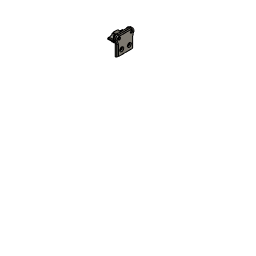
Insert Rig By Sadrita (Autodesk Fusion 360 archive; units mm, degrees)
design "Idler Plate M3"
Autodesk Fusion 360 part; units mm, degrees
sketch "Sketch1" plane through (10, 0, 0) normal (1, 0, 0) x (0, 1, 0)
  line L0 (3.15, 0) -> (10, 0)
  line L1 (10, 0) -> (10, 400)
  line L2 (10, 400) -> (3.15, 400)
  line L3 (3.15, 400) -> (3.15, 0) construction
  line L4 (10, 400) -> (-10, 400) construction
  line L5 (-10, 412) -> (10, 412) construction
  circle A0 centre (6, 412) radius 6
  circle A1 centre (6, 412) radius 2.8
  circle A2 centre (6, 412) radius 1.7
  circle A3 centre (0, 385) radius 2.75
  line L6 (0, 0) -> (0, 505.4699) construction
  line L7 (-10, 464.6221) -> (-10, 380.1585) construction
  circle A4 centre (-26, 412) radius 6
  circle A5 centre (-26, 412) radius 2.8
  circle A6 centre (-26, 412) radius 1.7
  circle A7 centre (6, 412) radius 7.5
  line L8 (10, 400) -> (13.1357, 409.6911)
  line L9 (10, 400) -> (10, 370)
  line L10 (10, 370) -> (-30, 370)
  line L11 (-30, 400) -> (-30, 370)
  line L12 (-30, 400) -> (-33.1357, 409.6911)
  circle A8 centre (-26, 412) radius 7.5
  line L13 (-26, 419.5) -> (6, 419.5)
  circle A9 centre (-20, 385) radius 2.75
  line L14 (2.5, 400) -> (-2.5, 400)
  line L15 (-2.5, 400) -> (-2.5, 370)
  line L16 (-2.5, 370) -> (2.5, 370)
  line L17 (2.5, 370) -> (2.5, 400)
  line L18 (2.5, 400) -> (-2.5, 370) construction
  line L19 (-2.5, 400) -> (2.5, 370) construction
  line L20 (10, 385) -> (-36.1637, 385) construction
  line L21 (-2.5, 391) -> (2.5, 391)
  line L22 (-2.5, 379) -> (2.5, 379)
  line L23 (3.15, 0) -> (10, 0)
  line L24 (10, 0) -> (10, 400)
  line L25 (10, 400) -> (3.15, 400)
  line L26 (3.15, 400) -> (3.15, 0)
  line L27 (-22.5, 370) -> (-22.5, 400)
  line L28 (-22.5, 400) -> (-17.5, 400)
  line L29 (-17.5, 370) -> (-22.5, 370)
  line L30 (-17.5, 400) -> (-17.5, 370)
  line L31 (-17.5, 391) -> (-22.5, 391)
  line L32 (-17.5, 379) -> (-22.5, 379)
  point P0 (6, 394.4653)
  point P1 (0, 385)
  dimension "d22" = 12
  dimension "d33" = 3.4
  dimension "d34" = 12
  dimension "d47" = 5.5
  dimension "d129" = 5.6
  dimension "d166" = 10
  dimension "d167" = 6
  dimension "d168" = 40
  dimension "d169" = 15
  dimension "d170" = 30
  dimension "d171" = 5
  dimension "d172" = 6
  dimension "d173" = 6
  constraint horizontal L4
  constraint coincident L1.end L2.start
  constraint concentric A0 A1
  constraint concentric A1 A2
  constraint vertical A0.centre P0
  constraint coincident L5 A0.centre
  constraint coincident L6.start origin
  constraint perpendicular L5 L6
  constraint vertical L7
  constraint symmetric A0 L7 A4
  constraint symmetric A1 L7 A5
  constraint symmetric A2 L7 A6
  constraint concentric A1 A7
  constraint coincident A7 L8.end
  constraint tangent A7 L8
  constraint coincident L1 L9.end
  constraint perpendicular L4 L9
  constraint perpendicular L9 L10
  constraint symmetric L1.end L7 L11.start
  constraint symmetric L7 A7 A8
  constraint symmetric L7 L8.end L12.end
  constraint symmetric L7 L9.end L10.end
  constraint coincident A8 L13.start
  constraint coincident A7 L13.end
  constraint tangent A7 L13
  constraint perpendicular L6 L13
  constraint coincident P1 L6
  constraint symmetric A3 L7 A9
  constraint horizontal L14
  constraint perpendicular L14 L15
  constraint parallel L14 L16
  constraint parallel L15 L17
  constraint coincident L4 L14.start
  constraint coincident L18 P1
  constraint coincident L19 P1
  constraint coincident P1 A3.centre
  constraint midpoint L9 L20.start
  constraint perpendicular L9 L20
  constraint coincident L10 L16.end
  constraint coincident L15 L21.start
  constraint coincident L17 L21.end
  constraint perpendicular L17 L21
  constraint coincident L15 L22.start
  constraint coincident L17 L22.end
  constraint perpendicular L17 L22
  constraint symmetric L7 L14.start L27.end
  constraint symmetric L7 L14.end L28.end
  constraint symmetric L7 L15.end L29.start
  constraint symmetric L7 L16.end L27.start
  constraint symmetric L7 L21.start L31.start
  constraint symmetric L7 L21.end L31.end
  constraint symmetric L7 L22.start L32.start
  constraint symmetric L7 L22.end L32.end
  measures "d22" diameter of A0
  measures "d33" diameter of A2
  measures "d34" distance of L4 L5
  measures "d47" diameter of A3
  measures "d129" diameter of A1
  measures "d166" distance of L6 L7
  measures "d167" distance of A0.centre L6
  measures "d168" distance of L9.end L10.end
  measures "d169" diameter of A7
  measures "d170" distance of L4 L10
  measures "d171" distance of L15.end L16.end
  measures "d172" distance of P1 L22
  measures "d173" distance of L20 L21
extrude "Extrude1" add sketch "Sketch1" along normal blind 7 contours L1 L2 L9 L10 L24 L25 L26 | L2 A3 A7 L8 L10 L11 L12 A8 L13 A9 L14 L15 L17 L25 L26 L27 L28 L30 | L10 L15 L16 L17 L22 | A3 L15 L17 L22 | A7 | L10 L27 L29 L30 L32 | A9 L27 L30 L32 | A3 L15 L17 L21 | A8 | L14 L15 L17 L21 | A9 L27 L30 L31 | L27 L28 L30 L31 | A0 | A1 | A4 | A5
extrude "Extrude3" add sketch "Sketch1" against normal blind 5.75 contours A0 | A1 | A2 | A4 | A5
extrude "Extrude6" cut sketch "Sketch1" along normal blind 2 from surface at -5.75 contours A0 | A4
extrude "Extrude7" cut sketch "Sketch1" along normal mid plane 28 contours A2
extrude "Extrude11" add sketch "Sketch1" against normal blind 3 contours L10 L15 L16 L17 L22 | L10 L27 L29 L30 L32 | L14 L15 L17 L21 | L27 L28 L30 L31
chamfer "Chamfer2" distance 3 angle 45 4 edges at (7, 0, 391) (7, 0, 379) (7, -20, 391) (7, -20, 379)
chamfer "Chamfer3" distance 1 angle 45 6 edges at (6.25, 0.406, 409.8303) (6.25, 3.3895, 413.0125) (10, 0.406, 409.8303) (10, -31.594, 409.8303) (6.25, -31.594, 409.8303) (6.25, -28.6105, 413.0125)
sketch "Sketch4" plane through (10, 0, 0) normal (-1, 0, 0) x (0, -1, 0)
  circle A0 centre (-6, 412) radius 7
  line L0 (17.5, 400) -> (22.5, 400)
  line L1 (22.5, 400) -> (22.5, 391)
  line L2 (17.5, 391) -> (17.5, 400)
  line L3 (22.5, 379) -> (22.5, 370)
  line L4 (22.5, 370) -> (30, 370)
  line L5 (30, 370) -> (30, 400)
  line L6 (30, 400) -> (33.1357, 409.6911)
  arc A1 (33.1357, 409.6911) -> (26, 419.5) centre (26, 412) ccw
  line L7 (26, 419.5) -> (-6, 419.5)
  arc A2 (-6, 419.5) -> (-13.1357, 409.6911) centre (-6, 412) ccw
  line L8 (-13.1357, 409.6911) -> (-10, 400)
  line L9 (-10, 400) -> (-10, 370)
  line L10 (-10, 370) -> (-2.5, 370)
  line L11 (-2.5, 370) -> (-2.5, 379)
  line L12 (2.5, 379) -> (2.5, 370)
  line L13 (2.5, 370) -> (17.5, 370)
  line L14 (17.5, 370) -> (17.5, 379)
  circle A3 centre (20, 385) radius 2.75
  circle A4 centre (0, 385) radius 2.75
  circle A5 centre (26, 412) radius 7
  line L15 (-10, 400) -> (30, 400)
  line L16 (-10.6471, 402) -> (30.6471, 402)
  circle A6 centre (-6, 412) radius 10
  circle A7 centre (26, 412) radius 10
  line L17 (3.1652, 408) -> (16.8348, 408)
  line L18 (22.5, 391) -> (17.5, 391)
  line L19 (-2.5, 391) -> (-2.5, 400)
  line L20 (-2.5, 400) -> (2.5, 400)
  line L21 (2.5, 400) -> (2.5, 391)
  line L22 (2.5, 391) -> (-2.5, 391)
  line L23 (-2.5, 379) -> (2.5, 379)
  line L24 (17.5, 379) -> (22.5, 379)
  dimension "d2" = 2
  dimension "d3" = 8
  constraint coincident L8.end L9.start
  constraint coincident L5.end L6.start
  constraint coincident L8 L16.start
  constraint coincident L6 L16.end
  constraint parallel L15 L16
  constraint concentric A0 A6
  constraint tangent L16 A6
  constraint concentric A1 A7
  constraint tangent L16 A7
  constraint coincident A6 L17.start
  constraint coincident A7 L17.end
  constraint horizontal L17
  measures "d2" distance of L15 L16
  measures "d3" distance of L15 L17
extrude "Extrude12" add sketch "Sketch4" along normal blind 20 contours L0 L6 L8 L15 L16 L20 | L16 A6 A7 L17
fillet "Fillet1" radius 1 4 edges at (0, 10.6471, 402) (0, -3.1652, 408) (0, -16.8348, 408) (0, -30.6471, 402)
sketch "Sketch5" plane through (17, 0, 0) normal (1, 0, 0) x (0, 1, 0)
  circle A0 centre (6, 412) radius 1.7
  circle A1 centre (-26, 412) radius 1.7
  circle A2 centre (0, 385) radius 2.75
  circle A3 centre (-20, 385) radius 2.75
  line L0 (-30, 370) -> (10, 370)
  line L1 (10, 370) -> (10, 400)
  line L2 (10, 400) -> (13.1357, 409.6911)
  arc A4 (13.1357, 409.6911) -> (6, 419.5) centre (6, 412) ccw
  line L3 (6, 419.5) -> (-26, 419.5)
  arc A5 (-26, 419.5) -> (-33.1357, 409.6911) centre (-26, 412) ccw
  line L4 (-33.1357, 409.6911) -> (-30, 400)
  line L5 (-30, 400) -> (-30, 370)
  line L6 (-27.631, 414.825) -> (-29.262, 412)
  line L7 (-29.262, 412) -> (-27.631, 409.175)
  line L8 (-27.631, 409.175) -> (-24.369, 409.175)
  line L9 (-24.369, 409.175) -> (-22.738, 412)
  line L10 (-22.738, 412) -> (-24.369, 414.825)
  line L11 (-24.369, 414.825) -> (-27.631, 414.825)
  line L12 (2.738, 412) -> (4.369, 409.175)
  line L13 (4.369, 409.175) -> (7.631, 409.175)
  line L14 (7.631, 409.175) -> (9.262, 412)
  line L15 (9.262, 412) -> (7.631, 414.825)
  line L16 (7.631, 414.825) -> (4.369, 414.825)
  line L17 (4.369, 414.825) -> (2.738, 412)
  circle A6 centre (-20, 385) radius 5.25
  circle A7 centre (0, 385) radius 5.25
  point P0 (-26, 412)
  point P1 (6, 412)
  dimension "d8" = 5.65
  dimension "d9" = 10.5
  constraint coincident P0 A1.centre
  constraint coincident A0.centre A4.centre
  constraint horizontal L11
  constraint horizontal L16
  constraint equal L11 L16
  constraint concentric A3 A6
  constraint concentric A2 A7
  constraint equal A6 A7
  measures "d8" distance of L13 L16
  measures "d9" diameter of A6
extrude "Extrude14" cut sketch "Sketch5" against normal blind 4 contours A6 | A7
extrude "Extrude13" cut sketch "Sketch5" against normal blind 5 contours L6 L7 L8 L9 L10 L11 | L12 L13 L14 L15 L16 L17
sketch "Sketch6" plane through (12, 0, 0) normal (1, 0, 0) x (0, 1, 0)
  circle A0 centre (-26, 412) radius 1.7
  line L0 (-24.369, 414.825) -> (-27.631, 414.825)
  line L1 (-27.631, 414.825) -> (-29.262, 412)
  line L2 (-29.262, 412) -> (-27.631, 409.175)
  line L3 (-27.631, 409.175) -> (-24.369, 409.175)
  line L4 (-24.369, 409.175) -> (-22.738, 412)
  line L5 (-22.738, 412) -> (-24.369, 414.825)
  circle A1 centre (6, 412) radius 1.7
  line L6 (4.369, 414.825) -> (2.738, 412)
  line L7 (2.738, 412) -> (4.369, 409.175)
  line L8 (4.369, 409.175) -> (7.631, 409.175)
  line L9 (7.631, 409.175) -> (9.262, 412)
  line L10 (9.262, 412) -> (7.631, 414.825)
  line L11 (7.631, 414.825) -> (4.369, 414.825)
  line L12 (-23.7195, 413.7) -> (-28.2805, 413.7)
  line L13 (-27.7, 413.7) -> (-27.7, 410.3)
  line L14 (-28.2805, 410.3) -> (-23.7195, 410.3)
  line L15 (-24.3, 410.3) -> (-24.3, 413.7)
  line L16 (-24.3, 413.7) -> (-27.7, 410.3) construction
  line L17 (-27.7, 413.7) -> (-24.3, 410.3) construction
  line L18 (8.2805, 413.7) -> (3.7195, 413.7)
  line L19 (4.3, 413.7) -> (4.3, 410.3)
  line L20 (3.7195, 410.3) -> (8.2805, 410.3)
  line L21 (7.7, 410.3) -> (7.7, 413.7)
  line L22 (7.7, 413.7) -> (4.3, 410.3) construction
  line L23 (4.3, 413.7) -> (7.7, 410.3) construction
  point P0 (-26, 412)
  point P1 (6, 412)
  constraint horizontal L12
  constraint perpendicular L12 L13
  constraint parallel L12 L14
  constraint parallel L13 L15
  constraint coincident L16 P0
  constraint coincident L17 P0
  constraint coincident P0 A0.centre
  constraint horizontal L18
  constraint perpendicular L18 L19
  constraint parallel L18 L20
  constraint parallel L19 L21
  constraint coincident L22 P1
  constraint coincident L23 P1
  constraint coincident P1 A1.centre
  constraint tangent A1 L18
  constraint tangent A1 L19
  constraint tangent A0 L12
  constraint tangent A0 L13
  constraint coincident L5 L12.start
  constraint coincident L15.end L12
  constraint coincident L1 L12.end
  constraint coincident L13.start L12
  constraint coincident L2 L14.start
  constraint coincident L13.end L14
  constraint coincident L4 L14.end
  constraint coincident L15.start L14
  constraint coincident L6 L18.end
  constraint coincident L19.start L18
  constraint coincident L10 L18.start
  constraint coincident L21.end L18
  constraint coincident L9 L20.end
  constraint coincident L21.start L20
  constraint coincident L7 L20.start
  constraint coincident L19.end L20
extrude "Extrude16" cut sketch "Sketch6" against normal blind 0.2 contours A0 L14 L15 | A0 L12 L15 | A0 L12 L13 | A0 L13 L14 | A1 L20 L21 | A1 L18 L21 | A1 L18 L19 | A1 L19 L20
extrude "Extrude15" add sketch "Sketch6" along normal blind 0.2 contours L0 L1 L5 L12 | L2 L3 L4 L14 | L6 L10 L11 L18 | L7 L8 L9 L20
sketch "Sketch7" plane through (13, 0, 0) normal (1, 0, 0) x (0, 1, 0)
  circle A0 centre (-20, 385) radius 2.75
  circle A1 centre (-20, 385) radius 5.25
  line L0 (-17.25, 387.75) -> (-22.75, 387.75)
  line L1 (-22.75, 389.4721) -> (-22.75, 380.5279)
  line L2 (-22.75, 382.25) -> (-17.25, 382.25)
  line L3 (-17.25, 380.5279) -> (-17.25, 389.4721)
  line L4 (-17.25, 387.75) -> (-22.75, 382.25) construction
  line L5 (-22.75, 387.75) -> (-17.25, 382.25) construction
  line L6 (2.75, 387.75) -> (-2.75, 387.75)
  line L7 (-2.75, 389.4721) -> (-2.75, 380.5279)
  line L8 (-2.75, 382.25) -> (2.75, 382.25)
  line L9 (2.75, 380.5279) -> (2.75, 389.4721)
  line L10 (2.75, 387.75) -> (-2.75, 382.25) construction
  line L11 (-2.75, 387.75) -> (2.75, 382.25) construction
  circle A2 centre (0, 385) radius 2.75
  circle A3 centre (0, 385) radius 2.75
  circle A4 centre (0, 385) radius 5.25
  point P0 (-20, 385)
  point P1 (0, 385)
  constraint horizontal L0
  constraint perpendicular L0 L1
  constraint parallel L0 L2
  constraint parallel L1 L3
  constraint coincident L4 P0
  constraint coincident L5 P0
  constraint coincident P0 A0.centre
  constraint horizontal L6
  constraint perpendicular L6 L7
  constraint parallel L6 L8
  constraint parallel L7 L9
  constraint coincident L10 P1
  constraint coincident L11 P1
  constraint tangent L6 A2
  constraint tangent L7 A2
  constraint tangent A0 L3
  constraint tangent A0 L0
  constraint tangent L9 A2
  constraint tangent L8 A2
  constraint coincident A1 L1.start
  constraint coincident L0.end L1
  constraint coincident A1 L1.end
  constraint coincident L2.start L1
  constraint coincident A1 L3.start
  constraint coincident L2.end L3
  constraint coincident A1 L3.end
  constraint coincident L0.start L3
  constraint coincident A4 L7.start
  constraint coincident L6.end L7
  constraint coincident A4 L7.end
  constraint coincident L8.start L7
  constraint coincident A4 L9.start
  constraint coincident L8.end L9
  constraint coincident A4 L9.end
  constraint coincident L6.start L9
extrude "Extrude18" cut sketch "Sketch7" against normal blind 0.2 contours A0 L2 L3 | A0 L0 L3 | A0 L0 L1 | A0 L1 L2 | L6 L9 A2 A3 | L6 L7 A2 A3 | L8 L9 A2 A3 | L7 L8 A2 A3
extrude "Extrude17" add sketch "Sketch7" along normal blind 0.2 contours A1 L3 | A1 L1 | L9 A4 | L7 A4
chamfer "Chamfer4" distance 1.5 distance2 3 7 edges at (17, -32.0649, 416.4121) (17, -31.5679, 404.8455) (17, 11.5679, 404.8455) (17, 12.0649, 416.4121) (17, -10, 419.5) (17, -30, 385) (17, 10, 385) measured on face at (17, -7.5417, 404.5155) measured on face at (17, -7.5417, 404.5155) measured on face at (17, -7.5417, 404.5155) measured on face at (17, -7.5417, 404.5155) measured on face at (17, -7.5417, 404.5155) measured on face at (17, -7.5417, 404.5155) measured on face at (17, -7.5417, 404.5155)
chamfer "Chamfer5" distance 3 distance2 5 1 edges at (17, -10, 370) measured on face at (17, -7.5417, 404.5155)
equation "d173 = d172"
named bodies: "M3 Idler Plate"
